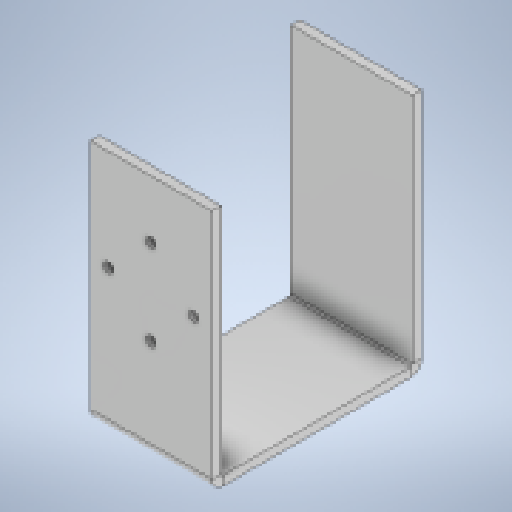
# Autodesk Inventor part: axis_7_top_frame
Saved by Autodesk Inventor 2025.2 (Build 292293000, 293)
## iProperties
Created: 2025-05-04
Part Number: axis_7_top_frame
Material: Aluminum 6061-AHC
Document SubType Name: Sheet Metal
Designer: User
Density: 2.7 g/cm^3
Sheet Metal Rule: Default_mm
Appearance: Aluminum - Dark
Author: User
Autodesk Inventor part; units mm, degrees
ref_plane "YZ Plane" through (0, 0, 0) normal (1, 0, 0) x (0, 1, 0)
ref_plane "XZ Plane" through (0, 0, 0) normal (0, 1, 0) x (-1, 0, 0)
ref_plane "XY Plane" through (0, 0, 0) normal (0, 0, 1) x (1, 0, 0)
sketch "Sketch1" plane through (0, 0, 0) normal (0, 1, 0) x (-1, 0, 0)
  line L0 (10, -15.715) -> (-10, -15.715)
  line L1 (-10, -15.715) -> (-10, 15.715)
  line L2 (-10, 15.715) -> (10, 15.715)
  line L3 (10, 15.715) -> (10, -15.715)
  point P0 (0, 0)
  dimension "d0" = 20
  dimension "d1" = 31.43
  dimension "d2" = 10
  dimension "d3" = 15.715
  measures "d0" distance of L0.start L0.end
  measures "d1" distance of L0.end L1.end
  measures "d2" distance from line of L3 point (0, 0)
  measures "d3" distance from line of point (0, 0) L0
extrude "Plate1" add sketch "Sketch1" along normal blind 1.5
sketch "Sketch2" plane through (10, 0, 17.215) normal (0, 0, -1) x (-1, 0, 0)
  line L0 (20, 0) -> (0, 0)
  line L1 (0, 0) -> (0, 40)
  line L2 (0, 40) -> (20, 40)
  line L3 (20, 40) -> (20, 0)
  constraints: 8 end point
edge flange "Flange1" height 40 angle 90 thickness 1.5 bend radius 0.31 thickness toward (0, 0, -1) relief tear relief width 1.5 relief depth 0.75 edges at (0, 1.5, 15.715) wall of the first edge with corners at (-10, 0, 17.215) (10, 0, 17.215) (10, 40, 17.215) (-10, 40, 17.215)
bend "Bend1"
corner "Corner1"
sketch "Sketch3" plane through (-10, 0, -17.215) normal (0, 0, 1) x (1, 0, 0)
  line L0 (20, 0) -> (0, 0)
  line L1 (0, 0) -> (0, 40)
  line L2 (0, 40) -> (20, 40)
  line L3 (20, 40) -> (20, 0)
  constraints: 8 end point
edge flange "Flange2" height 40 angle 90 thickness 1.5 bend radius 0.31 thickness toward (0, 0, 1) relief tear relief width 1.5 relief depth 0.75 edges at (0, 1.5, -15.715) wall of the first edge with corners at (10, 0, -17.215) (-10, 0, -17.215) (-10, 40, -17.215) (10, 40, -17.215)
bend "Bend2"
corner "Corner2"
sketch "Sketch4" plane through (10, 40, 15.715) normal (0, 0, -1) x (-1, 0, 0)
  line L0 (30.46, -23.2265) -> (30.46, -24.7935) projected
  line L1 (38.57, -15.71) -> (38.57, -17.31) projected
  circle A0 centre (3, -16.51) radius 0.7835 projected
  circle A1 centre (10, -9.51) radius 0.7835 projected
  line L2 (38.57, -15.71) -> (38.57, -17.31) projected
  line L3 (38.57, -15.71) -> (38.57, -17.31) projected
  line L4 (37.07, -17.31) -> (37.07, -15.71) projected
  line L5 (30.46, -23.2265) -> (30.46, -24.7935) projected
  circle A2 centre (10, -23.51) radius 0.7835 projected
  circle A3 centre (3, -16.51) radius 0.7835 projected
  circle A4 centre (17, -16.51) radius 0.7835 projected
  circle A5 centre (10, -9.51) radius 0.7835 projected
  point P0 (10, -40)
hole "Hole1" at (0, 16.49, 15.715) at (-7, 23.49, 15.715) at (0, 30.49, 15.715) at (7, 23.49, 15.715) direction (0, 0, 1) diameter 1.6 depth 1.5
sketch "Sketch5" plane through (0, 1.5, 0) normal (0, 1, 0) x (1, 0, 0)
  circle A0 centre (-7, -2.785) radius 0.7835 projected
  circle A1 centre (0, -9.785) radius 0.7835 projected
  circle A2 centre (7, -2.785) radius 0.7835 projected
  circle A3 centre (0, 4.215) radius 0.7835 projected
  point P0 (0, 0)
hole "Hole2" at (-7, 1.5, 2.785) at (0, 1.5, 9.785) at (7, 1.5, 2.785) at (0, 1.5, -4.215) direction (0, -1, 0) diameter 1.6 depth 1.5
equation "\"d30\" = Thickness"
equation "\"d37\" = Thickness"
equation "\"d4\" = Thickness"
equation "\"d5\" = BendReliefWidth"
equation "\"d6\" = BendReliefDepth"
equation "\"d7\" = MinimumRemnant"
equation "\"d8\" = TransitionRadius"
equation "\"d11\" = BendRadius"
equation "\"d12\" = CornerReliefSize"
equation "\"d13\" = GapSize"
equation "\"d14\" = JacobiRadiusSize"
equation "\"d15\" = BendReliefWidth"
equation "\"d16\" = BendReliefDepth"
equation "\"d17\" = MinimumRemnant"
equation "\"d18\" = TransitionRadius"
equation "\"d21\" = BendRadius"
equation "\"d22\" = CornerReliefSize"
equation "\"d23\" = GapSize"
equation "\"d24\" = JacobiRadiusSize"
equation "\"BendReliefWidth\" = Thickness"
equation "\"BendReliefDepth\" = 0.5 * Thickness"
equation "\"CornerReliefSize\" = 4 * Thickness"
equation "\"MinimumRemnant\" = 2 * Thickness"
equation "\"TransitionRadius\" = BendRadius"
equation "\"JacobiRadiusSize\" = BendRadius"
equation "\"GapSize\" = Thickness"
equation "\"Thickness\" = 1.5"
equation "\"BendRadius\" = 0.31"
body "Solid1"
